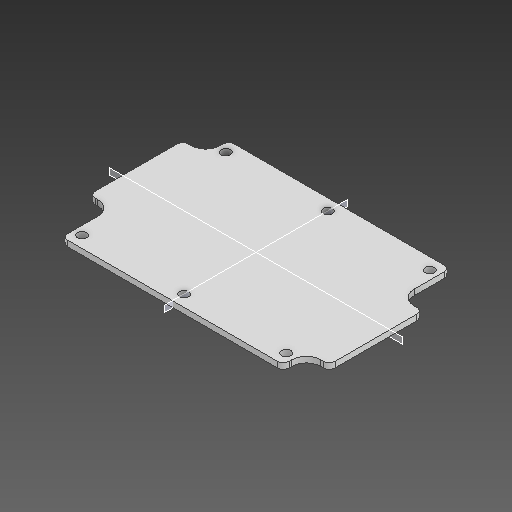
# Autodesk Inventor part: CH_01_0042_pcb_layout
Saved by Autodesk Inventor 2022 (Build 260153000, 153)
## iProperties
Created: 2022-07-25
Part Number: CH_01_0042_pcb_layout
Material: Generic
Document SubType Name: Modeling
Designer: Tomasz Krakowski
Density: 1 g/cm^3
Appearance: Default
Author: Tomasz Krakowski
Autodesk Inventor part; units mm, degrees
ref_plane "XZ Plane" through (0, 0, 0) normal (0, 1, 0) x (-1, 0, 0)
sketch "Sketch1" plane through (0, 0, 0) normal (0, 1, 0) x (-1, 0, 0)
  line L0 (-36.5, 29) -> (36.5, 29)
  line L1 (38.5, 27) -> (38.5, 16.5)
  line L2 (43.5, 11.5) -> (44.5, 11.5)
  line L3 (46.5, 9.5) -> (46.5, -19)
  line L4 (44.5, -21) -> (43.5, -21)
  line L5 (38.5, -26) -> (38.5, -27)
  line L6 (36.5, -29) -> (-36.5, -29)
  line L7 (0, 29) -> (0, -29) construction
  arc A0 (44.5, -21) -> (46.5, -19) centre (44.5, -19) ccw
  arc A1 (36.5, -29) -> (38.5, -27) centre (36.5, -27) ccw
  arc A2 (43.5, -21) -> (38.5, -26) centre (43.5, -26) ccw
  arc A3 (38.5, 16.5) -> (43.5, 11.5) centre (43.5, 16.5) ccw
  arc A4 (38.5, 27) -> (36.5, 29) centre (36.5, 27) ccw
  arc A5 (46.5, 9.5) -> (44.5, 11.5) centre (44.5, 9.5) ccw
  line L8 (-38.5, 27) -> (-38.5, 26)
  line L9 (-43.5, 21) -> (-44.5, 21)
  line L10 (-46.5, 19) -> (-46.5, -9.5)
  line L11 (-44.5, -11.5) -> (-43.5, -11.5)
  line L12 (-38.5, -16.5) -> (-38.5, -27)
  arc A6 (-36.5, 29) -> (-38.5, 27) centre (-36.5, 27) ccw
  arc A7 (-44.5, 21) -> (-46.5, 19) centre (-44.5, 19) ccw
  arc A8 (-46.5, -9.5) -> (-44.5, -11.5) centre (-44.5, -9.5) ccw
  arc A9 (-38.5, -27) -> (-36.5, -29) centre (-36.5, -27) ccw
  arc A10 (-43.5, 21) -> (-38.5, 26) centre (-43.5, 26) ccw
  arc A11 (-38.5, -16.5) -> (-43.5, -11.5) centre (-43.5, -16.5) ccw
  point P0 (0, 0)
  point P1 (38.5, 29)
  point P2 (38.5, -21)
  point P3 (38.5, -29)
  point P4 (0, 0)
  point P5 (-38.5, -11.5)
  dimension "d0" = 8
  dimension "d2" = 8
  dimension "d3" = 2
  dimension "d4" = 5
  dimension "d5" = 17.5
  dimension "d6" = 5
  dimension "d7" = 2
  dimension "d8" = 58
  dimension "d9" = 8
  dimension "d10" = 17.5
  dimension "d11" = 8
  dimension "d12" = 93
  dimension "d13" = 2
  dimension "d14" = 5
  constraints: 26 end point, 24 point on circle, 24 tangent, 12 centre point, 11 point on line, 8 perpendicular, 6 equal radius, 3 midpoint, 2 vertical, 1 coincident, 1 horizontal
  measures "d0" distance between parallel lines of L3 L5
  measures "d2" distance between parallel lines of L6 L4
  measures "d3" radius of A0
  measures "d4" radius of A2
  measures "d5" distance from line of L2 point (38.5, 29)
  measures "d6" radius of A3
  measures "d7" radius of A4
  measures "d8" distance between parallel lines of L6 L0
  measures "d9" distance between parallel lines of L12 L10
  measures "d10" distance between parallel lines of L6 L11
  measures "d11" distance between parallel lines of L0 L9
  measures "d12" distance between parallel lines of L3 L10
  measures "d13" radius of A6
  measures "d14" radius of A10
extrude "Extrusion1" add sketch "Sketch1" along normal blind 2
sketch "Sketch2" plane through (0, 2, 0) normal (0, 1, 0) x (1, 0, 0)
  line L0 (35.5, 25) -> (-35.5, 25) construction
  line L1 (-35.5, 25) -> (-35.5, -25) construction
  line L2 (-35.5, -25) -> (35.5, -25) construction
  line L3 (35.5, -25) -> (35.5, 25) construction
  line L4 (35.5, 25) -> (-35.5, -25) construction
  line L5 (-35.5, 25) -> (35.5, -25) construction
  point P0 (0, 0)
  point P1 (0, -25)
  point P2 (0, 25)
  point P3 (0, 25)
  point P4 (0, -25)
  dimension "d17" = 35.5
  dimension "d18" = 50
  constraints: 12 end point, 5 coincident, 4 midpoint, 2 parallel, 1 horizontal, 1 perpendicular
  measures "d17" distance from line of point (0, -25) L3
  measures "d18" distance of L2.end L0.start
hole "Hole1" at (0, 2, 25) at (-35.5, 2, 25) at (-35.5, 2, -25) at (0, 2, -25) at (35.5, 2, 25) at (35.5, 2, -25) direction (0, -1, 0) diameter 3.2 depth 7.5
equation "\"d2\" = d0"
equation "\"d6\" = d4"
equation "\"d7\" = d3"
equation "\"d9\" = d0"
equation "\"d10\" = d5"
equation "\"d11\" = d0"
equation "\"d13\" = d3"
equation "\"d14\" = d4"
body "Solid1"
